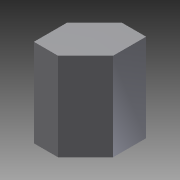
# Autodesk Inventor part: MotorCarrier
Saved by Autodesk Inventor 2012 SP2 (Build 160219200, 219)
## iProperties
Created: 2014-02-06
Part Number: MotorCarrier
Material: Default
Document SubType Name: Modeling
Designer: 1
Density: 1 g/cm^3
Author: 1
Autodesk Inventor part; units mm, degrees
ref_plane "YZ Plane" through (0, 0, 0) normal (1, 0, 0) x (0, 1, 0)
ref_plane "XZ Plane" through (0, 0, 0) normal (0, 1, 0) x (-1, 0, 0)
ref_plane "XY Plane" through (0, 0, 0) normal (0, 0, 1) x (1, 0, 0)
sketch "Sketch1" plane through (0, 0, 0) normal (0, 0, 1) x (1, 0, 0)
  line L0 (105.0559, -3.8299) -> (47.0396, -3.8299)
  line L1 (47.0396, -3.8299) -> (47.0396, -56.241)
  line L2 (47.0396, -56.241) -> (105.0559, -56.241)
  line L3 (105.0559, -56.241) -> (105.0559, -3.8299)
  point P0 (0, 0)
  constraints: 8 end point, 2 parallel, 1 horizontal, 1 perpendicular
extrude "Extrusion1" add sketch "Sketch1" along normal blind 46.0375 and the other way blind 23.8252
chamfer "Chamfer1" distance 31.75 angle 45 1 edges at (47.0396, -30.0355, -23.8252)
chamfer "Chamfer2" distance 31.75 angle 45 1 edges at (105.0559, -30.0355, 46.0375)
sketch "Sketch2" plane through (0, 0, 46.0375) normal (0, 0, 1) x (1, 0, 0)
  circle A0 centre (63.8131, -28.5354) radius 10
  point P0 (0, 0)
  dimension "d11" = 20
  constraints: 1 centre point
  measures "d11" diameter of A0
extrude "Extrusion2" cut sketch "Sketch2" against normal through all
body "Solid1"
